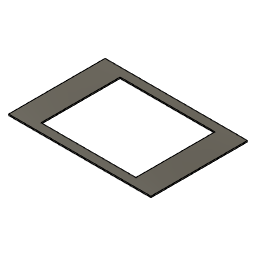
Frame V2 v8 (Autodesk Fusion 360 archive; units mm, degrees)
design "Top Bed"
Autodesk Fusion 360 part; units mm, degrees
sketch "Sketch1" plane through (0, 0, 0) normal (0, 0, 1) x (1, 0, 0)
  line L0 (-180, 122) -> (180, 122)
  line L1 (180, 122) -> (180, -122)
  line L2 (180, -122) -> (-180, -122)
  line L3 (-180, -122) -> (-180, 122)
  line L4 (-180, 122) -> (180, -122) construction
  line L5 (180, 122) -> (-180, -122) construction
  line L6 (-150, 100) -> (150, 100)
  line L7 (150, 100) -> (150, -100)
  line L8 (150, -100) -> (-150, -100)
  line L9 (-150, -100) -> (-150, 100)
  line L10 (-150, 100) -> (150, -100) construction
  line L11 (150, 100) -> (-150, -100) construction
  dimension "d1" = 244
  dimension "d2" = 360
  dimension "d3" = 300
  dimension "d4" = 200
  constraint horizontal L0
  constraint perpendicular L0 L1
  constraint parallel L0 L2
  constraint parallel L1 L3
  constraint coincident L4 origin
  constraint coincident L5 origin
  constraint horizontal L6
  constraint perpendicular L6 L7
  constraint parallel L6 L8
  constraint parallel L7 L9
  constraint coincident L10 origin
  constraint coincident L11 origin
  measures "d1" distance of L0.end L1.end
  measures "d2" distance of L1 L3
  measures "d3" distance of L7.end L8.end
  measures "d4" distance of L6.end L7.end
extrude "Extrude1" add sketch "Sketch1" along normal blind 3
extrude "Extrude2" add 1 faces at (-150, -33.3333, 1) along direction (1, 0, 0) blind 30
extrude "Extrude3" add 1 faces at (150, 33.3333, 1) along direction (-1, 0, 0) blind 30
sketch "Sketch2" plane through (0, 0, 3) normal (0, 0, 1) x (-1, 0, 0)
  line L0 (-120, 100) -> (120, 100)
  line L1 (120, 100) -> (120, -100)
  line L2 (120, -100) -> (-120, -100)
  line L3 (-120, -100) -> (-120, 100)
  line L4 (180, 122) -> (-180, 122)
  line L5 (-180, 122) -> (-180, -122)
  line L6 (-180, -122) -> (180, -122)
  line L7 (180, -122) -> (180, 122)

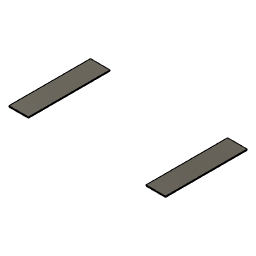
design "Stair Climber Bed"
Autodesk Fusion 360 part; units mm, degrees
sketch "Sketch1" plane through (0, 0, 0) normal (0, 0, 1) x (1, 0, 0)
  line L0 (240, 125) -> (-240, 125)
  line L1 (-240, 125) -> (-240, -125)
  line L2 (-240, -125) -> (240, -125)
  line L3 (240, -125) -> (240, 125)
  line L4 (240, 125) -> (-240, -125) construction
  line L5 (-240, 125) -> (240, -125) construction
  dimension "d1" = 480
  dimension "d2" = 250
  constraint horizontal L0
  constraint perpendicular L0 L1
  constraint parallel L0 L2
  constraint parallel L1 L3
  constraint coincident L4 origin
  constraint coincident L5 origin
  measures "d1" distance of L1.end L2.end
  measures "d2" distance of L0.end L1.end
extrude "Extrude1" add sketch "Sketch1" along normal blind 3 makes body 1
sketch "Sketch2" plane through (0, 0, 3) normal (0, 0, 1) x (-1, 0, 0)
  line L0 (-240, 125) -> (-240, -125)
  line L1 (-240, -125) -> (240, -125)
  line L2 (240, -125) -> (240, 125)
  line L3 (240, 125) -> (-240, 125)
  line L4 (0, 0) -> (210, 0) construction
  line L5 (0, 0) -> (-210, 0) construction
  line L6 (210, 0) -> (210, -125) construction
  line L7 (210, 0) -> (210, 125) construction
  line L8 (-210, 0) -> (-210, -125) construction
  line L9 (-210, 0) -> (-210, 125) construction
  dimension "d5" = 210
  dimension "d6" = 210
  constraint coincident L4.start L5.start
  constraint perpendicular L0 L4
  constraint perpendicular L0 L5
  constraint coincident L1 L6.end
  constraint perpendicular L1 L6
  constraint coincident L3 L7.end
  constraint perpendicular L3 L7
  constraint coincident L1 L8.end
  constraint perpendicular L1 L8
  constraint coincident L3 L9.end
  constraint perpendicular L3 L9
  measures "d5" distance of L4.start L4.end
  measures "d6" distance of L4.start L5.end
sketch "Sketch3" plane through (0, 0, 3) normal (0, 0, 1) x (-1, 0, 0)
  line L0 (210, 125) -> (180, 125) construction
  line L1 (180, 125) -> (180, -125) construction
  line L2 (180, -125) -> (210, -125) construction
  line L3 (210, -125) -> (210, 125) construction
  line L4 (-210, 125) -> (-180, 125) construction
  line L5 (-180, 125) -> (-180, -125) construction
  line L6 (-180, -125) -> (-210, -125) construction
  line L7 (-210, -125) -> (-210, 125) construction
  line L8 (180, -125) -> (-180, -125)
  line L9 (-180, -125) -> (-180, 125)
  line L10 (-180, 125) -> (180, 125)
  line L11 (180, 125) -> (180, -125)
  dimension "d7" = 30
  dimension "d8" = 250
  dimension "d9" = 30
  dimension "d10" = 250
  constraint horizontal L0
  constraint vertical L1
  constraint horizontal L2
  constraint vertical L3
  constraint horizontal L4
  constraint vertical L5
  constraint horizontal L6
  constraint vertical L7
  constraint horizontal L8
  constraint vertical L9
  constraint horizontal L10
  constraint vertical L11
  measures "d7" distance of L0.start L0.end
  measures "d8" distance of L0.start L2.end
  measures "d9" distance of L4.start L4.end
  measures "d10" distance of L4.start L6.end
extrude "Extrude2" cut sketch "Sketch3" against normal blind 20 bodies 1 makes body 2 at (200, 41.6667, 0)
sketch "Sketch4" plane through (0, 0, 3) normal (0, 0, 1) x (-1, 0, 0)
  line L0 (180, 125) -> (180, -125)
  line L1 (180, -125) -> (240, -125)
  line L2 (240, -125) -> (240, 125)
  line L3 (240, 125) -> (180, 125)

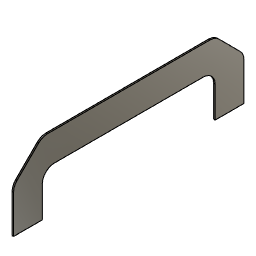
design "Side frame"
Autodesk Fusion 360 part; units mm, degrees
sketch "Sketch1" plane through (0, 0, 0) normal (1, 0, 0) x (0, 1, 0)
  line L0 (180, 75) -> (-180, 75)
  line L1 (-240, 15) -> (-240, -75)
  line L2 (240, -75) -> (240, 15)
  line L3 (-240, -75) -> (-180, -75)
  line L4 (-180, -75) -> (-180, 75)
  line L5 (-240, 15) -> (-240, -75)
  line L6 (240, -75) -> (180, -75)
  line L7 (180, -75) -> (180, 75)
  line L8 (240, 15) -> (240, -75)
  line L9 (-180, 75) -> (180, 75)
  line L10 (240, 15) -> (-240, 15)
  line L11 (-240, 15) -> (-180, 75)
  line L12 (240, 15) -> (180, 75)
  line L13 (-240, -75) -> (-180, -75)
  line L14 (180, -75) -> (240, -75)
  line L15 (194.2857, 60.7143) -> (48, 15) construction
  line L16 (-194.2857, 60.7143) -> (-48, 15) construction
  line L17 (180, -56.25) -> (240, -75) construction
  line L18 (0, 55) -> (5, 55)
  line L19 (5, 35) -> (0, 35)
  line L20 (5, 65) -> (10, 65)
  line L21 (10, 65) -> (10, 25)
  line L22 (10, 25) -> (5, 25)
  line L23 (0, 75) -> (0, 55)
  line L24 (0, 35) -> (0, 15)
  line L25 (5, 25) -> (5, 35)
  line L26 (5, 55) -> (5, 65)
  dimension "d1" = 480
  dimension "d3" = 60
  dimension "d5" = 60
  constraint horizontal L0
  constraint perpendicular L0 L1
  constraint parallel L0 L13
  constraint parallel L1 L2
  constraint coincident origin L15
  constraint coincident origin L16
  constraint horizontal L3
  constraint vertical L4
  constraint vertical L5
  constraint horizontal L6
  constraint vertical L7
  constraint vertical L8
  constraint horizontal L9
  constraint horizontal L10
  constraint coincident L12 L15.start
  constraint coincident L11 L16.start
  constraint collinear L13 L14
  constraint coincident L7 L17.start
  constraint collinear L16 L17
  constraint coincident L10 L16.end
  constraint coincident L10 L15.end
  constraint midpoint L0 L23.start
  constraint midpoint L10 L24.end
  constraint horizontal L18
  constraint horizontal L19
  constraint horizontal L20
  constraint vertical L21
  constraint horizontal L22
  constraint vertical L25
  constraint collinear L23 L24
  constraint collinear L25 L26
  measures "d1" distance of L1.end L2.start
  measures "d3" distance of L1.end L3.end
  measures "d5" distance of L2.start L6.end
extrude "Extrude1" add sketch "Sketch1" along normal blind 3
sketch "Sketch2" plane through (0, 0, 0) normal (-1, 0, 0) x (0, -1, 0)
  line L0 (-180, -75) -> (-180, 15)
  line L1 (-180, 15) -> (180, 15)
  line L2 (180, 15) -> (180, -75)
  line L3 (180, -75) -> (240, -75)
  line L4 (240, -75) -> (240, 15)
  line L5 (240, 15) -> (180, 75)
  line L6 (180, 75) -> (-180, 75)
  line L7 (-180, 75) -> (-240, 15)
  line L8 (-240, 15) -> (-240, -75)
  line L9 (-240, -75) -> (-180, -75)
  line L10 (0, 55) -> (5, 55)
  line L11 (5, 35) -> (0, 35)
  line L12 (5, 65) -> (10, 65)
  line L13 (10, 65) -> (10, 25)
  line L14 (10, 25) -> (5, 25)
  line L15 (5, 25) -> (5, 35)
  line L16 (5, 55) -> (5, 65)
  line L17 (0, 55) -> (0, 75)
  line L18 (0, 35) -> (0, 15)
  constraint horizontal L10
  constraint horizontal L11
  constraint horizontal L12
  constraint vertical L13
  constraint horizontal L14
  constraint vertical L15
  constraint collinear L15 L16
  constraint midpoint L6 L17.end
  constraint perpendicular L10 L17
  constraint midpoint L1 L18.end
  constraint perpendicular L1 L18
fillet "Fillet1" radius 25 2 edges at (1.5, -180, 15) (1.5, 180, 15)
fillet "Fillet2" radius 25 4 edges at (1.5, -240, 15) (1.5, -180, 75) (1.5, 180, 75) (1.5, 240, 15)
sketch "Sketch3" plane through (3, 0, 0) normal (1, 0, 0) x (0, 1, 0)
  arc A0 (240, 4.6447) -> (232.6777, 22.3223) centre (215, 4.6447) ccw
  line L0 (232.6777, 22.3223) -> (187.3223, 67.6777)
  arc A1 (187.3223, 67.6777) -> (169.6447, 75) centre (169.6447, 50) ccw
  line L1 (169.6447, 75) -> (-169.6447, 75)
  arc A2 (-169.6447, 75) -> (-187.3223, 67.6777) centre (-169.6447, 50) ccw
  line L2 (-187.3223, 67.6777) -> (-232.6777, 22.3223)
  arc A3 (-232.6777, 22.3223) -> (-240, 4.6447) centre (-215, 4.6447) ccw
  line L3 (-240, 4.6447) -> (-240, -75)
  line L4 (-240, -75) -> (-180, -75)
  line L5 (-180, -75) -> (-180, -10)
  arc A4 (-155, 15) -> (-180, -10) centre (-155, -10) ccw
  line L6 (-155, 15) -> (155, 15)
  arc A5 (180, -10) -> (155, 15) centre (155, -10) ccw
  line L7 (180, -10) -> (180, -75)
  line L8 (180, -75) -> (240, -75)
  line L9 (240, -75) -> (240, 4.6447)
